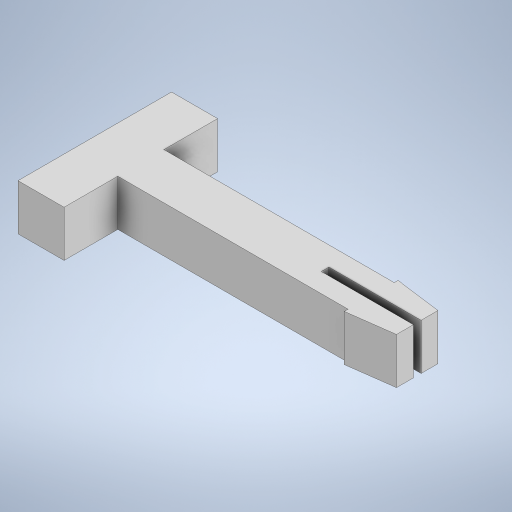
# Autodesk Inventor part: 插銷A
Saved by Autodesk Inventor 2024 (Build 280153000, 153)
## iProperties
Created: 2024-04-14
Part Number: 插銷A
Material: 一般
Document SubType Name: Modeling
Designer: USER
Density: 1 g/cm^3
Appearance: 預設
Author: USER
Autodesk Inventor part; units mm, degrees
ref_plane "YZ Plane" through (0, 0, 0) normal (1, 0, 0) x (0, 1, 0)
ref_plane "XZ Plane" through (0, 0, 0) normal (0, 1, 0) x (-1, 0, 0)
ref_plane "XY Plane" through (0, 0, 0) normal (0, 0, 1) x (1, 0, 0)
sketch "草圖1" plane through (0, 0, 0) normal (0, 1, 0) x (-1, 0, 0)
  line L0 (15, 1.5) -> (0, 1.5)
  line L1 (0, 1.5) -> (0, -1.5)
  line L2 (0, -1.5) -> (15, -1.5)
  line L3 (15, -1.5) -> (15, 1.5)
  line L4 (18, 5) -> (15, 5)
  line L5 (15, 5) -> (15, -5)
  line L6 (15, -5) -> (18, -5)
  line L7 (18, -5) -> (18, 5)
  line L8 (0, 0) -> (15, 0)
  line L9 (0, 1.5) -> (0, 1.75)
  line L10 (0, 1.35) -> (-3, 1.35)
  line L11 (0, 1.75) -> (-3, 1.35)
  line L12 (-3, 1.35) -> (-3, 0.25)
  line L13 (-3, 0.25) -> (0, 0.25)
  line L14 (0, -1.5) -> (0, -1.75)
  line L15 (0, -1.35) -> (-3, -1.35)
  line L16 (0, -1.75) -> (-3, -1.35)
  line L17 (-3, -1.35) -> (-3, -0.25)
  line L18 (-3, -0.25) -> (0, -0.25)
  line L19 (0, 0.25) -> (3, 0.25)
  line L20 (3, 0.25) -> (3, -0.25)
  line L21 (3, -0.25) -> (0, -0.25)
  point P0 (0, -0.25)
  dimension "d0" = 3
  dimension "d1" = 15
  dimension "d2" = 10
  dimension "d3" = 3
  dimension "d4" = 0.25
  dimension "d5" = 3
  dimension "d6" = 0.15
  dimension "d7" = 1.1
  dimension "d10" = 3
  constraints: 44 end point, 6 parallel, 5 symmetric about line, 4 perpendicular, 3 horizontal, 3 midpoint, 2 point on line, 2 vertical, 1 coincident, 1 collinear
  measures "d0" distance of L0.end L1.end
  measures "d1" distance of L1.end L2.end
  measures "d2" distance of L6.end L4.start
  measures "d3" distance of L5.end L6.end
  measures "d4" distance of L0.end L9.end
  measures "d5" distance of L10.start L10.end
  measures "d6" distance of L10.start L0.end
  measures "d7" distance of L10.end L12.end
  measures "d10" distance of L13.end L19.end
extrude "擠出1" add sketch "草圖1" along normal blind 3 contours L3 L8 L20 L19 L1 L0 | L5 L4 L7 L6 L3 | L1 L10 L11 L9 | L3 L2 L1 L21 L20 L8 | L1 L13 L12 L10 | L14 L16 L15 L1 | L15 L17 L18 L1
